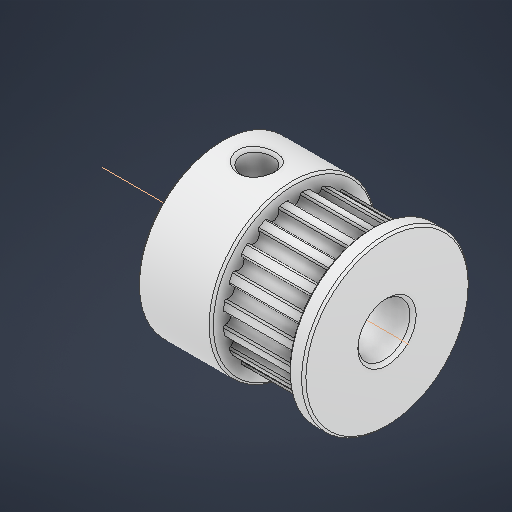
# Autodesk Inventor part: GT2Pulley_z20
Saved by Autodesk Inventor 2025.2 (Build 292293000, 293)
## iProperties
Created: 2025-05-15
Part Number: GT2Pulley_z20
Material: Generic
Document SubType Name: Modeling
Designer: Tiago
Density: 1 g/cm^3
Appearance: Aluminum - Dark
Author: Tiago
Autodesk Inventor part; units mm, degrees
ref_plane "YZ Plane" through (0, 0, 0) normal (1, 0, 0) x (0, 1, 0)
sketch "Sketch1" plane through (0, 0, 0) normal (0, 0, 1) x (1, 0, 0)
  line L0 (0, 2.5) -> (0, 8)
  line L1 (0, 8) -> (7.1, 8)
  line L2 (7.1, 8) -> (7.1, 6.11)
  line L3 (7.1, 6.11) -> (14.5, 6.11)
  line L4 (14.5, 6.11) -> (14.5, 8)
  line L5 (14.5, 8) -> (16, 8)
  line L6 (16, 8) -> (16, 2.5)
  line L7 (16, 0) -> (0, 0)
  line L8 (0, 2.5) -> (16, 2.5)
  dimension "L" = 16
  dimension "d1" = 7.1
  dimension "DE" = 16
  dimension "d3" = 12.22
  dimension "d4" = 7.4
  dimension "d5" = 16
  dimension "Bore" = 5
  constraints: 18 end point, 7 perpendicular, 2 vertical alignment, 1 horizontal, 1 vertical
  measures "L" distance of L7.start L7.end
  measures "d1" distance between parallel lines of L0 L2
  measures "DE" diameter of L1 L7
  measures "d3" diameter of L3 L7
  measures "d4" distance between parallel lines of L4 L2
  measures "d5" diameter of L5 L7
  measures "Bore" diameter of L8 L7
revolve "Revolution1" add sketch "Sketch1" angle 360 about axis through (16, 0, 0) along (-1, 0, 0)
sketch "Sketch3" plane through (7.1, 0, 0) normal (1, 0, 0) x (0, 0, -1)
  line L0 (0, 0) -> (0, 8.9731) construction
  line L1 (0, 0) -> (1.4779, 9.3313) construction
  line L2 (0, 0) -> (2.089, 9.3456) construction
  line L3 (0, 0) -> (2.8787, 8.8598) construction
  circle A0 centre (0, 0) radius 6.11
  circle A1 centre (0, 0) radius 6.665 construction
  arc A2 (1.5337, 6.5162) -> (1.4227, 6.7109) centre (1.3916, 6.5641) ccw
  arc A3 (1.5337, 6.5162) -> (1.8881, 5.811) centre (2.0596, 6.3388) ccw
  arc A4 (0.7207, 6.822) -> (0.555, 6.6712) centre (0.705, 6.6729) ccw
  arc A5 (0, 6.11) -> (0.555, 6.6712) centre (0, 6.665) ccw
  arc A6 (0, 6.86) -> (2.1199, 6.5242) centre (0, 0) ccw construction
  arc A7 (1.4227, 6.7109) -> (0.7207, 6.822) centre (0, 0) ccw
  point P0 (0, 6.11)
  dimension "d11" = 12.22
  dimension "d12" = 0.555
  dimension "d13" = 0.555
  dimension "d8" = 9
  dimension "d9" = 18
  dimension "d10" = 3.6
  dimension "d16" = 0.3
  dimension "d17" = 0.555
  dimension "d18" = 0.15
  dimension "d19" = 6.86
  constraints: 12 point on circle, 8 end point, 6 centre point, 5 symmetric about line, 3 point on line, 2 tangent, 1 coincident, 1 vertical, 8 other
  measures "d8" angle of L0 L1
  measures "d9" angle of L0 L3
  measures "d10" angle of L1 L2
  measures "d16" diameter of A2
  measures "d17" radius of A3
  measures "d18" radius of A2
  measures "d19" radius of A7
extrude "Extrusion1" add sketch "Sketch3" along normal up to surface (7.4 mm away) contours A0 A5 A4 A7 A2 A3
pattern_circular "Circular Pattern1" count 20 over 360 about axis through (-10, 0, 0) along (1, 0, 0) of "Extrusion1"
ref_plane "Work Plane1" through (3.55, 8, 0) normal (0, 1, 0) x (-1, 0, 0)
sketch "Sketch4" plane through (3.55, 8, 0) normal (0, 1, 0) x (-1, 0, 0)
  circle A0 centre (0.05, 0) radius 1.5
  line L0 (3.55, -8) -> (3.55, 8) projected
  point P0 (3.55, 0)
  dimension "d25" = 3
  dimension "d26" = 3.5
  constraints: 1 centre point, 1 horizontal alignment
  measures "d25" diameter of A0
  measures "d26" distance from line of A0.centre L0
extrude "Extrusion2" cut sketch "Sketch4" against normal up to surface round surface about axis through (8, 0, 0) along (-1, 0, 0) radius 2.5 far side no
ref_plane "Work Plane2" through (3.55, 0, -8) normal (0, 0, 1) x (1, 0, 0)
sketch "Sketch5" plane through (3.55, 0, -8) normal (0, 0, 1) x (1, 0, 0)
  circle A0 centre (-0.05, 0) radius 1.5
  line L0 (-3.55, 8) -> (-3.55, -8) projected
  point P0 (-3.55, 0)
  dimension "Furo" = 3
  dimension "d30" = 3.5
  constraints: 1 centre point
  measures "Furo" diameter of A0
  measures "d30" distance from line of A0.centre L0
extrude "Extrusion3" cut sketch "Sketch5" along normal up to surface round surface about axis through (8, 0, 0) along (-1, 0, 0) radius 2.5 far side no
chamfer "Chamfer1" distance 0.2 angle 45 4 edges at (16, -8, 0) (14.5, -8, 0) (7.1, -8, 0) (0, -8, 0)
chamfer "Chamfer2" distance 0.3 angle 45 6 edges at (3.5002, 7.8581, -1.5) (3.4999, 7.8581, 1.5) (3.3675, -1.4941, -7.8592) (3.5015, 1.5, -7.8581) (16, -2.5, 0) (0, -2.5, 0)
equation "\"d5\" = DE"
equation "\"d25\" = Furo"
body "Solid1"
